Autodesk Fusion 360 part; units mm, degrees
(part 4 of 6)
  spline S7 degree 5 poles (100.0499, 27.0485) (100.0462, 27.0591) (100.039, 27.0805) (100.028, 27.1124) (100.0132, 27.1549) (99.9945, 27.2079) (99.9756, 27.2608) (99.9566, 27.3135) (99.9373, 27.366) (99.9178, 27.4184) (99.8981, 27.4707) (99.8782, 27.5228) (99.858, 27.5747) (99.8377, 27.6265) (99.8172, 27.6781) (99.7964, 27.7296) (99.7755, 27.7809) (99.7543, 27.832) (99.7329, 27.883) (99.7113, 27.9338) (99.6895, 27.9844) (99.6674, 28.0349) (99.6452, 28.0852) (99.6227, 28.1353) (99.6, 28.1852) (99.5771, 28.235) (99.554, 28.2846) (99.5307, 28.334) (99.5071, 28.3832) (99.4833, 28.4322) (99.4593, 28.481) (99.435, 28.5297) (99.4105, 28.5781) (99.3858, 28.6263) (99.3609, 28.6744) (99.3357, 28.7222) (99.3103, 28.7698) (99.2846, 28.8173) (99.2587, 28.8645) (99.2326, 28.9115) (99.2062, 28.9582) (99.1796, 29.0048) (99.1527, 29.0511) (99.1256, 29.0972) (99.0982, 29.143) (99.0706, 29.1886) (99.0427, 29.234) (99.0146, 29.2791) (98.9862, 29.324) (98.9575, 29.3686) (98.9286, 29.4129) (98.8993, 29.457) (98.8698, 29.5007) (98.84, 29.5442) (98.8098, 29.5873) (98.7794, 29.6302) (98.7487, 29.6728) (98.7177, 29.7152) (98.6865, 29.7572) (98.655, 29.7989) (98.623, 29.8402) (98.5906, 29.8811) (98.5578, 29.9214) (98.5245, 29.9612) (98.4907, 30.0006) (98.4567, 30.0397) (98.4225, 30.0785) (98.388, 30.1171) (98.3533, 30.1553) (98.3179, 30.1928) (98.2816, 30.2292) (98.2515, 30.2572) (98.2282, 30.2774) (98.2123, 30.2904) (98.2043, 30.2969) knots -1 -1 -1 -1 -1 -1 -0.98571429 -0.97142857 -0.95714286 -0.94285714 -0.92857143 -0.91428571 -0.9 -0.88571429 -0.87142857 -0.85714286 -0.84285714 -0.82857143 -0.81428571 -0.8 -0.78571429 -0.77142857 -0.75714286 -0.74285714 -0.72857143 -0.71428571 -0.7 -0.68571429 -0.67142857 -0.65714286 -0.64285714 -0.62857143 -0.61428571 -0.6 -0.58571429 -0.57142857 -0.55714286 -0.54285714 -0.52857143 -0.51428571 -0.5 -0.48571429 -0.47142857 -0.45714286 -0.44285714 -0.42857143 -0.41428571 -0.4 -0.38571429 -0.37142857 -0.35714286 -0.34285714 -0.32857143 -0.31428571 -0.3 -0.28571429 -0.27142857 -0.25714286 -0.24285714 -0.22857143 -0.21428571 -0.2 -0.18571429 -0.17142857 -0.15714286 -0.14285714 -0.12857143 -0.11428571 -0.1 -0.08571429 -0.07142857 -0.05714286 -0.04285714 -0.02857143 -0.01428571 0 0 0 0 0 0
  line L7 (98.2043, 30.2969) -> (97.816, 30.6089)
  arc A17 (97.7326, 31.303) -> (97.816, 30.6089) centre (98.1293, 30.9987) ccw
  arc A18 (97.7326, 31.303) -> (98.4247, 32.2557) centre (79.882, 45) ccw
  arc A19 (99.1106, 32.3908) -> (98.4247, 32.2557) centre (98.8368, 31.9725) ccw
  line L8 (99.1106, 32.3908) -> (99.5274, 32.118)
  spline S8 degree 5 poles (99.5274, 32.118) (99.536, 32.1123) (99.5534, 32.1013) (99.5797, 32.0854) (99.6156, 32.0654) (99.6615, 32.0421) (99.7081, 32.0201) (99.7552, 31.9988) (99.8025, 31.978) (99.85, 31.9574) (99.8977, 31.9371) (99.9456, 31.9172) (99.9938, 31.8978) (100.0423, 31.8791) (100.0911, 31.8609) (100.1403, 31.8433) (100.1897, 31.8261) (100.2393, 31.8094) (100.2892, 31.7931) (100.3392, 31.777) (100.3893, 31.7614) (100.4397, 31.746) (100.4902, 31.7311) (100.541, 31.7165) (100.5919, 31.7023) (100.643, 31.6885) (100.6943, 31.675) (100.7458, 31.6619) (100.7974, 31.6491) (100.8492, 31.6366) (100.9011, 31.6244) (100.9531, 31.6125) (101.0053, 31.6009) (101.0577, 31.5897) (101.1102, 31.5788) (101.1628, 31.5681) (101.2156, 31.5578) (101.2685, 31.5478) (101.3215, 31.538) (101.3746, 31.5286) (101.4279, 31.5194) (101.4813, 31.5105) (101.5348, 31.5019) (101.5884, 31.4936) (101.6422, 31.4856) (101.6961, 31.4778) (101.75, 31.4703) (101.8041, 31.4631) (101.8583, 31.4562) (101.9126, 31.4495) (101.967, 31.4431) (102.0215, 31.4369) (102.0761, 31.4311) (102.1308, 31.4254) (102.1856, 31.4201) (102.2405, 31.415) (102.2955, 31.4101) (102.3506, 31.4055) (102.4058, 31.4012) (102.461, 31.3971) (102.5164, 31.3933) (102.5718, 31.3897) (102.6274, 31.3864) (102.683, 31.3833) (102.7387, 31.3805) (102.7945, 31.3779) (102.8503, 31.3755) (102.9063, 31.3734) (102.9623, 31.3715) (103.0184, 31.3699) (103.0746, 31.3685) (103.1196, 31.3676) (103.1533, 31.3671) (103.1759, 31.3667) (103.1872, 31.3666) knots 0 0 0 0 0 0 0.01428571 0.02857143 0.04285714 0.05714286 0.07142857 0.08571429 0.1 0.11428571 0.12857143 0.14285714 0.15714286 0.17142857 0.18571429 0.2 0.21428571 0.22857143 0.24285714 0.25714286 0.27142857 0.28571429 0.3 0.31428571 0.32857143 0.34285714 0.35714286 0.37142857 0.38571429 0.4 0.41428571 0.42857143 0.44285714 0.45714286 0.47142857 0.48571429 0.5 0.51428571 0.52857143 0.54285714 0.55714286 0.57142857 0.58571429 0.6 0.61428571 0.62857143 0.64285714 0.65714286 0.67142857 0.68571429 0.7 0.71428571 0.72857143 0.74285714 0.75714286 0.77142857 0.78571429 0.8 0.81428571 0.82857143 0.84285714 0.85714286 0.87142857 0.88571429 0.9 0.91428571 0.92857143 0.94285714 0.95714286 0.97142857 0.98571429 1 1 1 1 1 1
  arc A20 (103.1872, 31.3666) -> (103.8806, 32.628) centre (79.882, 45) ccw
  spline S9 degree 5 poles (103.8806, 32.628) (103.8745, 32.6374) (103.8621, 32.6563) (103.8435, 32.6845) (103.8186, 32.722) (103.7874, 32.7687) (103.7559, 32.8152) (103.7243, 32.8615) (103.6926, 32.9076) (103.6607, 32.9535) (103.6286, 32.9992) (103.5964, 33.0447) (103.564, 33.09) (103.5314, 33.1351) (103.4987, 33.18) (103.4658, 33.2247) (103.4327, 33.2692) (103.3995, 33.3134) (103.3661, 33.3575) (103.3325, 33.4013) (103.2988, 33.4449) (103.2649, 33.4883) (103.2308, 33.5315) (103.1966, 33.5745) (103.1622, 33.6172) (103.1277, 33.6597) (103.0929, 33.7019) (103.058, 33.744) (103.023, 33.7858) (102.9877, 33.8273) (102.9523, 33.8687) (102.9167, 33.9097) (102.881, 33.9506) (102.845, 33.9911) (102.8089, 34.0315) (102.7726, 34.0715) (102.7362, 34.1113) (102.6995, 34.1509) (102.6627, 34.1902) (102.6257, 34.2292) (102.5886, 34.2679) (102.5512, 34.3064) (102.5137, 34.3446) (102.4759, 34.3825) (102.438, 34.4201) (102.3999, 34.4574) (102.3616, 34.4944) (102.3231, 34.5311) (102.2845, 34.5675) (102.2456, 34.6036) (102.2065, 34.6393) (102.1673, 34.6747) (102.1278, 34.7098) (102.0881, 34.7444) (102.0481, 34.7787) (102.008, 34.8127) (101.9677, 34.8463) (101.9272, 34.8796) (101.8865, 34.9126) (101.8455, 34.9451) (101.8043, 34.9772) (101.7628, 35.0087) (101.7209, 35.0396) (101.6788, 35.0699) (101.6363, 35.0997) (101.5936, 35.129) (101.5508, 35.1581) (101.5079, 35.1869) (101.4647, 35.2152) (101.4211, 35.2428) (101.3769, 35.2691) (101.3408, 35.2887) (101.3132, 35.3024) (101.2946, 35.3111) (101.2852, 35.3154) knots -1 -1 -1 -1 -1 -1 -0.98571429 -0.97142857 -0.95714286 -0.94285714 -0.92857143 -0.91428571 -0.9 -0.88571429 -0.87142857 -0.85714286 -0.84285714 -0.82857143 -0.81428571 -0.8 -0.78571429 -0.77142857 -0.75714286 -0.74285714 -0.72857143 -0.71428571 -0.7 -0.68571429 -0.67142857 -0.65714286 -0.64285714 -0.62857143 -0.61428571 -0.6 -0.58571429 -0.57142857 -0.55714286 -0.54285714 -0.52857143 -0.51428571 -0.5 -0.48571429 -0.47142857 -0.45714286 -0.44285714 -0.42857143 -0.41428571 -0.4 -0.38571429 -0.37142857 -0.35714286 -0.34285714 -0.32857143 -0.31428571 -0.3 -0.28571429 -0.27142857 -0.25714286 -0.24285714 -0.22857143 -0.21428571 -0.2 -0.18571429 -0.17142857 -0.15714286 -0.14285714 -0.12857143 -0.11428571 -0.1 -0.08571429 -0.07142857 -0.05714286 -0.04285714 -0.02857143 -0.01428571 0 0 0 0 0 0
  line L9 (101.2852, 35.3154) -> (100.8315, 35.5211)
  arc A21 (100.5781, 36.1726) -> (100.8315, 35.5211) centre (101.038, 35.9765) ccw
  arc A22 (100.5781, 36.1726) -> (101.0116, 37.2674) centre (79.882, 45) ccw
  arc A23 (101.6423, 37.5689) -> (101.0116, 37.2674) centre (101.4811, 37.0956) ccw
  line L10 (101.6423, 37.5689) -> (102.1139, 37.4083)
  spline S10 degree 5 poles (102.1139, 37.4083) (102.1236, 37.405) (102.1431, 37.3986) (102.1726, 37.3897) (102.2124, 37.3793) (102.2626, 37.3682) (102.3132, 37.3584) (102.3641, 37.3495) (102.4151, 37.3411) (102.4662, 37.333) (102.5175, 37.3252) (102.5688, 37.3178) (102.6203, 37.311) (102.6719, 37.3049) (102.7238, 37.2995) (102.7758, 37.2946) (102.8279, 37.2903) (102.8801, 37.2865) (102.9325, 37.283) (102.9849, 37.28) (103.0374, 37.2772) (103.09, 37.2749) (103.1426, 37.273) (103.1954, 37.2715) (103.2483, 37.2704) (103.3012, 37.2697) (103.3543, 37.2695) (103.4074, 37.2695) (103.4605, 37.2699) (103.5138, 37.2707) (103.5671, 37.2718) (103.6205, 37.2733) (103.6739, 37.275) (103.7274, 37.2772) (103.781, 37.2796) (103.8346, 37.2824) (103.8883, 37.2855) (103.942, 37.289) (103.9958, 37.2927) (104.0496, 37.2968) (104.1035, 37.3012) (104.1574, 37.3059) (104.2114, 37.3108) (104.2654, 37.3161) (104.3195, 37.3217) (104.3736, 37.3276) (104.4277, 37.3337) (104.4819, 37.3402) (104.5361, 37.347) (104.5903, 37.354) (104.6446, 37.3613) (104.699, 37.3689) (104.7533, 37.3768) (104.8077, 37.385) (104.8621, 37.3934) (104.9165, 37.4021) (104.971, 37.4111) (105.0255, 37.4203) (105.08, 37.4299) (105.1346, 37.4397) (105.1892, 37.4497) (105.2437, 37.46) (105.2984, 37.4706) (105.353, 37.4815) (105.4077, 37.4926) (105.4623, 37.5039) (105.517, 37.5155) (105.5717, 37.5274) (105.6264, 37.5395) (105.6812, 37.5519) (105.7359, 37.5646) (105.7797, 37.5749) (105.8126, 37.5827) (105.8345, 37.588) (105.8455, 37.5906) knots 0 0 0 0 0 0 0.01428571 0.02857143 0.04285714 0.05714286 0.07142857 0.08571429 0.1 0.11428571 0.12857143 0.14285714 0.15714286 0.17142857 0.18571429 0.2 0.21428571 0.22857143 0.24285714 0.25714286 0.27142857 0.28571429 0.3 0.31428571 0.32857143 0.34285714 0.35714286 0.37142857 0.38571429 0.4 0.41428571 0.42857143 0.44285714 0.45714286 0.47142857 0.48571429 0.5 0.51428571 0.52857143 0.54285714 0.55714286 0.57142857 0.58571429 0.6 0.61428571 0.62857143 0.64285714 0.65714286 0.67142857 0.68571429 0.7 0.71428571 0.72857143 0.74285714 0.75714286 0.77142857 0.78571429 0.8 0.81428571 0.82857143 0.84285714 0.85714286 0.87142857 0.88571429 0.9 0.91428571 0.92857143 0.94285714 0.95714286 0.97142857 0.98571429 1 1 1 1 1 1
  arc A24 (105.8455, 37.5906) -> (106.2035, 38.9849) centre (79.882, 45) ccw
  spline S11 degree 5 poles (106.2035, 38.9849) (106.1951, 38.9925) (106.1785, 39.0077) (106.1535, 39.0304) (106.12, 39.0605) (106.0781, 39.098) (106.0361, 39.1352) (105.994, 39.1722) (105.9518, 39.2089) (105.9095, 39.2455) (105.867, 39.2817) (105.8245, 39.3178) (105.7818, 39.3536) (105.7391, 39.3892) (105.6962, 39.4246) (105.6532, 39.4597) (105.6101, 39.4945) (105.567, 39.5291) (105.5237, 39.5635) (105.4803, 39.5976) (105.4367, 39.6315) (105.3931, 39.6651) (105.3494, 39.6984) (105.3056, 39.7315) (105.2616, 39.7643) (105.2176, 39.7969) (105.1734, 39.8292) (105.1292, 39.8612) (105.0848, 39.893) (105.0403, 39.9245) (104.9958, 39.9557) (104.9511, 39.9867) (104.9063, 40.0173) (104.8614, 40.0477) (104.8164, 40.0778) (104.7713, 40.1075) (104.7261, 40.137) (104.6807, 40.1662) (104.6353, 40.1951) (104.5898, 40.2237) (104.5441, 40.252) (104.4984, 40.28) (104.4525, 40.3076) (104.4066, 40.3349) (104.3605, 40.3619) (104.3143, 40.3885) (104.268, 40.4149) (104.2216, 40.4408) (104.1751, 40.4665) (104.1285, 40.4918) (104.0818, 40.5167) (104.0349, 40.5412) (103.988, 40.5653) (103.9409, 40.589) (103.8937, 40.6123) (103.8464, 40.6352) (103.7989, 40.6578) (103.7514, 40.68) (103.7038, 40.7018) (103.656, 40.7231) (103.6082, 40.7439) (103.5601, 40.7641) (103.5119, 40.7836) (103.4635, 40.8025) (103.415, 40.8208) (103.3663, 40.8386) (103.3176, 40.8561) (103.2689, 40.8733) (103.22, 40.89) (103.1709, 40.9059) (103.1216, 40.9203) (103.0817, 40.9303) (103.0516, 40.9368) (103.0314, 40.9406) (103.0213, 40.9424) knots -1 -1 -1 -1 -1 -1 -0.98571429 -0.97142857 -0.95714286 -0.94285714 -0.92857143 -0.91428571 -0.9 -0.88571429 -0.87142857 -0.85714286 -0.84285714 -0.82857143 -0.81428571 -0.8 -0.78571429 -0.77142857 -0.75714286 -0.74285714 -0.72857143 -0.71428571 -0.7 -0.68571429 -0.67142857 -0.65714286 -0.64285714 -0.62857143 -0.61428571 -0.6 -0.58571429 -0.57142857 -0.55714286 -0.54285714 -0.52857143 -0.51428571 -0.5 -0.48571429 -0.47142857 -0.45714286 -0.44285714 -0.42857143 -0.41428571 -0.4 -0.38571429 -0.37142857 -0.35714286 -0.34285714 -0.32857143 -0.31428571 -0.3 -0.28571429 -0.27142857 -0.25714286 -0.24285714 -0.22857143 -0.21428571 -0.2 -0.18571429 -0.17142857 -0.15714286 -0.14285714 -0.12857143 -0.11428571 -0.1 -0.08571429 -0.07142857 -0.05714286 -0.04285714 -0.02857143 -0.01428571 0 0 0 0 0 0
  line L11 (103.0213, 40.9424) -> (102.5307, 41.0288)
  arc A25 (102.1232, 41.5969) -> (102.5307, 41.0288) centre (102.6174, 41.5212) ccw
  arc A26 (102.1232, 41.5969) -> (102.2707, 42.7651) centre (79.882, 45) ccw
  arc A27 (102.8067, 43.2139) -> (102.2707, 42.7651) centre (102.7683, 42.7154) ccw
  line L12 (102.8067, 43.2139) -> (103.3034, 43.1756)
  spline S12 degree 5 poles (103.3034, 43.1756) (103.3136, 43.1748) (103.3342, 43.1735) (103.3649, 43.1723) (103.406, 43.1721) (103.4574, 43.1738) (103.5089, 43.1769) (103.5604, 43.181) (103.6119, 43.1855) (103.6634, 43.1903) (103.715, 43.1955) (103.7665, 43.2012) (103.8181, 43.2074) (103.8696, 43.2143) (103.9212, 43.2219) (103.9728, 43.2302) (104.0243, 43.239) (104.0759, 43.2482) (104.1274, 43.2579) (104.1789, 43.2679) (104.2305, 43.2784) (104.282, 43.2892) (104.3335, 43.3004) (104.385, 43.3121) (104.4364, 43.3242) (104.4879, 43.3367) (104.5393, 43.3496) (104.5908, 43.3629) (104.6422, 43.3765) (104.6935, 43.3905) (104.7449, 43.4048) (104.7962, 43.4195) (104.8476, 43.4345) (104.8989, 43.4499) (104.9501, 43.4656) (105.0014, 43.4816) (105.0526, 43.498) (105.1038, 43.5147) (105.1549, 43.5317) (105.206, 43.549) (105.2571, 43.5667) (105.3082, 43.5846) (105.3592, 43.6029) (105.4103, 43.6214) (105.4612, 43.6403) (105.5122, 43.6594) (105.5631, 43.6789) (105.6139, 43.6986) (105.6648, 43.7186) (105.7156, 43.7389) (105.7663, 43.7595) (105.8171, 43.7804) (105.8677, 43.8015) (105.9184, 43.823) (105.969, 43.8447) (106.0196, 43.8666) (106.0701, 43.8889) (106.1206, 43.9114) (106.171, 43.9342) (106.2214, 43.9572) (106.2718, 43.9806) (106.3221, 44.0041) (106.3723, 44.028) (106.4226, 44.052) (106.4727, 44.0764) (106.5229, 44.101) (106.573, 44.1258) (106.623, 44.151) (106.673, 44.1763) (106.7229, 44.2019) (106.7728, 44.2278) (106.8127, 44.2486) (106.8426, 44.2644) (106.8625, 44.275) (106.8724, 44.2803) knots 0 0 0 0 0 0 0.01428571 0.02857143 0.04285714 0.05714286 0.07142857 0.08571429 0.1 0.11428571 0.12857143 0.14285714 0.15714286 0.17142857 0.18571429 0.2 0.21428571 0.22857143 0.24285714 0.25714286 0.27142857 0.28571429 0.3 0.31428571 0.32857143 0.34285714 0.35714286 0.37142857 0.38571429 0.4 0.41428571 0.42857143 0.44285714 0.45714286 0.47142857 0.48571429 0.5 0.51428571 0.52857143 0.54285714 0.55714286 0.57142857 0.58571429 0.6 0.61428571 0.62857143 0.64285714 0.65714286 0.67142857 0.68571429 0.7 0.71428571 0.72857143 0.74285714 0.75714286 0.77142857 0.78571429 0.8 0.81428571 0.82857143 0.84285714 0.85714286 0.87142857 0.88571429 0.9 0.91428571 0.92857143 0.94285714 0.95714286 0.97142857 0.98571429 1 1 1 1 1 1
  arc A28 (106.8724, 44.2803) -> (106.8724, 45.7197) centre (79.882, 45) ccw
  spline S13 degree 5 poles (106.8724, 45.7197) (106.8625, 45.725) (106.8426, 45.7356) (106.8127, 45.7514) (106.7728, 45.7722) (106.7229, 45.7981) (106.673, 45.8237) (106.623, 45.849) (106.573, 45.8742) (106.5229, 45.899) (106.4727, 45.9236) (106.4226, 45.948) (106.3723, 45.972) (106.3221, 45.9959) (106.2718, 46.0194) (106.2214, 46.0428) (106.171, 46.0658) (106.1206, 46.0886) (106.0701, 46.1111) (106.0196, 46.1334) (105.969, 46.1553) (105.9184, 46.177) (105.8677, 46.1985) (105.8171, 46.2196) (105.7663, 46.2405) (105.7156, 46.2611) (105.6648, 46.2814) (105.6139, 46.3014) (105.5631, 46.3211) (105.5122, 46.3406) (105.4612, 46.3597) (105.4103, 46.3786) (105.3592, 46.3971) (105.3082, 46.4154) (105.2571, 46.4333) (105.206, 46.451) (105.1549, 46.4683) (105.1038, 46.4853) (105.0526, 46.502) (105.0014, 46.5184) (104.9501, 46.5344) (104.8989, 46.5501) (104.8476, 46.5655) (104.7962, 46.5805) (104.7449, 46.5952) (104.6935, 46.6095) (104.6422, 46.6235) (104.5908, 46.6371) (104.5393, 46.6504) (104.4879, 46.6633) (104.4364, 46.6758) (104.385, 46.6879) (104.3335, 46.6996) (104.282, 46.7108) (104.2305, 46.7216) (104.1789, 46.7321) (104.1274, 46.7421) (104.0759, 46.7518) (104.0243, 46.761) (103.9728, 46.7698) (103.9212, 46.7781) (103.8696, 46.7857) (103.8181, 46.7926) (103.7665, 46.7988) (103.715, 46.8045) (103.6634, 46.8097) (103.6119, 46.8145) (103.5604, 46.819) (103.5089, 46.8231) (103.4574, 46.8262) (103.406, 46.8279) (103.3649, 46.8277) (103.3342, 46.8265) (103.3136, 46.8252) (103.3034, 46.8244) knots -1 -1 -1 -1 -1 -1 -0.98571429 -0.97142857 -0.95714286 -0.94285714 -0.92857143 -0.91428571 -0.9 -0.88571429 -0.87142857 -0.85714286 -0.84285714 -0.82857143 -0.81428571 -0.8 -0.78571429 -0.77142857 -0.75714286 -0.74285714 -0.72857143 -0.71428571 -0.7 -0.68571429 -0.67142857 -0.65714286 -0.64285714 -0.62857143 -0.61428571 -0.6 -0.58571429 -0.57142857 -0.55714286 -0.54285714 -0.52857143 -0.51428571 -0.5 -0.48571429 -0.47142857 -0.45714286 -0.44285714 -0.42857143 -0.41428571 -0.4 -0.38571429 -0.37142857 -0.35714286 -0.34285714 -0.32857143 -0.31428571 -0.3 -0.28571429 -0.27142857 -0.25714286 -0.24285714 -0.22857143 -0.21428571 -0.2 -0.18571429 -0.17142857 -0.15714286 -0.14285714 -0.12857143 -0.11428571 -0.1 -0.08571429 -0.07142857 -0.05714286 -0.04285714 -0.02857143 -0.01428571 0 0 0 0 0 0
  line L13 (103.3034, 46.8244) -> (102.8067, 46.7861)
  arc A29 (102.2707, 47.2349) -> (102.8067, 46.7861) centre (102.7683, 47.2846) ccw
  arc A30 (102.2707, 47.2349) -> (102.1232, 48.4031) centre (79.882, 45) ccw
  arc A31 (102.5307, 48.9712) -> (102.1232, 48.4031) centre (102.6174, 48.4788) ccw
  line L14 (102.5307, 48.9712) -> (103.0213, 49.0576)
  spline S14 degree 5 poles (103.0213, 49.0576) (103.0314, 49.0594) (103.0516, 49.0632) (103.0817, 49.0697) (103.1216, 49.0797) (103.1709, 49.0941) (103.22, 49.11) (103.2689, 49.1267) (103.3176, 49.1439) (103.3663, 49.1614) (103.415, 49.1792) (103.4635, 49.1975) (103.5119, 49.2164) (103.5601, 49.2359) (103.6082, 49.2561) (103.656, 49.2769) (103.7038, 49.2982) (103.7514, 49.32) (103.7989, 49.3422) (103.8464, 49.3648) (103.8937, 49.3877) (103.9409, 49.411) (103.988, 49.4347) (104.0349, 49.4588) (104.0818, 49.4833) (104.1285, 49.5082) (104.1751, 49.5335) (104.2216, 49.5592) (104.268, 49.5851) (104.3143, 49.6115) (104.3605, 49.6381) (104.4066, 49.6651) (104.4525, 49.6924) (104.4984, 49.72) (104.5441, 49.748) (104.5898, 49.7763) (104.6353, 49.8049) (104.6807, 49.8338) (104.7261, 49.863) (104.7713, 49.8925) (104.8164, 49.9222) (104.8614, 49.9523) (104.9063, 49.9827) (104.9511, 50.0133) (104.9958, 50.0443) (105.0403, 50.0755) (105.0848, 50.107) (105.1292, 50.1388) (105.1734, 50.1708) (105.2176, 50.2031) (105.2616, 50.2357) (105.3056, 50.2685) (105.3494, 50.3016) (105.3931, 50.3349) (105.4367, 50.3685) (105.4803, 50.4024) (105.5237, 50.4365) (105.567, 50.4709) (105.6101, 50.5055) (105.6532, 50.5403) (105.6962, 50.5754) (105.7391, 50.6108) (105.7818, 50.6464) (105.8245, 50.6822) (105.867, 50.7183) (105.9095, 50.7545) (105.9518, 50.7911) (105.994, 50.8278) (106.0361, 50.8648) (106.0781, 50.902) (106.12, 50.9395) (106.1535, 50.9696) (106.1785, 50.9923) (106.1951, 51.0075) (106.2035, 51.0151) knots 0 0 0 0 0 0 0.01428571 0.02857143 0.04285714 0.05714286 0.07142857 0.08571429 0.1 0.11428571 0.12857143 0.14285714 0.15714286 0.17142857 0.18571429 0.2 0.21428571 0.22857143 0.24285714 0.25714286 0.27142857 0.28571429 0.3 0.31428571 0.32857143 0.34285714 0.35714286 0.37142857 0.38571429 0.4 0.41428571 0.42857143 0.44285714 0.45714286 0.47142857 0.48571429 0.5 0.51428571 0.52857143 0.54285714 0.55714286 0.57142857 0.58571429 0.6 0.61428571 0.62857143 0.64285714 0.65714286 0.67142857 0.68571429 0.7 0.71428571 0.72857143 0.74285714 0.75714286 0.77142857 0.78571429 0.8 0.81428571 0.82857143 0.84285714 0.85714286 0.87142857 0.88571429 0.9 0.91428571 0.92857143 0.94285714 0.95714286 0.97142857 0.98571429 1 1 1 1 1 1
  arc A32 (106.2035, 51.0151) -> (105.8455, 52.4094) centre (79.882, 45) ccw
  spline S15 degree 5 poles (105.8455, 52.4094) (105.8345, 52.412) (105.8126, 52.4173) (105.7797, 52.4251) (105.7359, 52.4354) (105.6812, 52.4481) (105.6264, 52.4605) (105.5717, 52.4726) (105.517, 52.4845) (105.4623, 52.4961) (105.4077, 52.5074) (105.353, 52.5185) (105.2984, 52.5294) (105.2437, 52.54) (105.1892, 52.5503) (105.1346, 52.5603) (105.08, 52.5701) (105.0255, 52.5797) (104.971, 52.5889) (104.9165, 52.5979) (104.8621, 52.6066) (104.8077, 52.615) (104.7533, 52.6232) (104.699, 52.6311) (104.6446, 52.6387) (104.5903, 52.646) (104.5361, 52.653) (104.4819, 52.6598) (104.4277, 52.6663) (104.3736, 52.6724) (104.3195, 52.6783) (104.2654, 52.6839) (104.2114, 52.6892) (104.1574, 52.6941) (104.1035, 52.6988) (104.0496, 52.7032) (103.9958, 52.7073) (103.942, 52.711) (103.8883, 52.7145) (103.8346, 52.7176) (103.781, 52.7204) (103.7274, 52.7228) (103.6739, 52.725) (103.6205, 52.7267) (103.5671, 52.7282) (103.5138, 52.7293) (103.4605, 52.7301) (103.4074, 52.7305) (103.3543, 52.7305) (103.3012, 52.7303) (103.2483, 52.7296) (103.1954, 52.7285) (103.1426, 52.727) (103.09, 52.7251) (103.0374, 52.7228) (102.9849, 52.72) (102.9325, 52.717) (102.8801, 52.7135) (102.8279, 52.7097) (102.7758, 52.7054) (102.7238, 52.7005) (102.6719, 52.6951) (102.6203, 52.689) (102.5688, 52.6822) (102.5175, 52.6748) (102.4662, 52.667) (102.4151, 52.6589) (102.3641, 52.6505) (102.3132, 52.6416) (102.2626, 52.6318) (102.2124, 52.6207) (102.1726, 52.6103) (102.1431, 52.6014) (102.1236, 52.595) (102.1139, 52.5917) knots -1 -1 -1 -1 -1 -1 -0.98571429 -0.97142857 -0.95714286 -0.94285714 -0.92857143 -0.91428571 -0.9 -0.88571429 -0.87142857 -0.85714286 -0.84285714 -0.82857143 -0.81428571 -0.8 -0.78571429 -0.77142857 -0.75714286 -0.74285714 -0.72857143 -0.71428571 -0.7 -0.68571429 -0.67142857 -0.65714286 -0.64285714 -0.62857143 -0.61428571 -0.6 -0.58571429 -0.57142857 -0.55714286 -0.54285714 -0.52857143 -0.51428571 -0.5 -0.48571429 -0.47142857 -0.45714286 -0.44285714 -0.42857143 -0.41428571 -0.4 -0.38571429 -0.37142857 -0.35714286 -0.34285714 -0.32857143 -0.31428571 -0.3 -0.28571429 -0.27142857 -0.25714286 -0.24285714 -0.22857143 -0.21428571 -0.2 -0.18571429 -0.17142857 -0.15714286 -0.14285714 -0.12857143 -0.11428571 -0.1 -0.08571429 -0.07142857 -0.05714286 -0.04285714 -0.02857143 -0.01428571 0 0 0 0 0 0
  line L15 (102.1139, 52.5917) -> (101.6423, 52.4311)
  arc A33 (101.0116, 52.7326) -> (101.6423, 52.4311) centre (101.4811, 52.9044) ccw
  arc A34 (101.0116, 52.7326) -> (100.5781, 53.8274) centre (79.882, 45) ccw
  arc A35 (100.8315, 54.4789) -> (100.5781, 53.8274) centre (101.038, 54.0235) ccw
  line L16 (100.8315, 54.4789) -> (101.2852, 54.6846)
  spline S16 degree 5 poles (101.2852, 54.6846) (101.2946, 54.6889) (101.3132, 54.6976) (101.3408, 54.7113) (101.3769, 54.7309) (101.4211, 54.7572) (101.4647, 54.7848) (101.5079, 54.8131) (101.5508, 54.8419) (101.5936, 54.871) (101.6363, 54.9003) (101.6788, 54.9301) (101.7209, 54.9604) (101.7628, 54.9913) (101.8043, 55.0228) (101.8455, 55.0549) (101.8865, 55.0874) (101.9272, 55.1204) (101.9677, 55.1537) (102.008, 55.1873) (102.0481, 55.2213) (102.0881, 55.2556) (102.1278, 55.2902) (102.1673, 55.3253) (102.2065, 55.3607) (102.2456, 55.3964) (102.2845, 55.4325) (102.3231, 55.4689) (102.3616, 55.5056) (102.3999, 55.5426) (102.438, 55.5799) (102.4759, 55.6175) (102.5137, 55.6554) (102.5512, 55.6936) (102.5886, 55.7321) (102.6257, 55.7708) (102.6627, 55.8098) (102.6995, 55.8491) (102.7362, 55.8887) (102.7726, 55.9285) (102.8089, 55.9685) (102.845, 56.0089) (102.881, 56.0494) (102.9167, 56.0903) (102.9523, 56.1313) (102.9877, 56.1727) (103.023, 56.2142) (103.058, 56.256) (103.0929, 56.2981) (103.1277, 56.3403) (103.1622, 56.3828) (103.1966, 56.4255) (103.2308, 56.4685) (103.2649, 56.5117) (103.2988, 56.5551) (103.3325, 56.5987) (103.3661, 56.6425) (103.3995, 56.6866) (103.4327, 56.7308) (103.4658, 56.7753) (103.4987, 56.82) (103.5314, 56.8649) (103.564, 56.91) (103.5964, 56.9553) (103.6286, 57.0008) (103.6607, 57.0465) (103.6926, 57.0924) (103.7243, 57.1385) (103.7559, 57.1848) (103.7874, 57.2313) (103.8186, 57.278) (103.8435, 57.3155) (103.8621, 57.3437) (103.8745, 57.3626) (103.8806, 57.372) knots 0 0 0 0 0 0 0.01428571 0.02857143 0.04285714 0.05714286 0.07142857 0.08571429 0.1 0.11428571 0.12857143 0.14285714 0.15714286 0.17142857 0.18571429 0.2 0.21428571 0.22857143 0.24285714 0.25714286 0.27142857 0.28571429 0.3 0.31428571 0.32857143 0.34285714 0.35714286 0.37142857 0.38571429 0.4 0.41428571 0.42857143 0.44285714 0.45714286 0.47142857 0.48571429 0.5 0.51428571 0.52857143 0.54285714 0.55714286 0.57142857 0.58571429 0.6 0.61428571 0.62857143 0.64285714 0.65714286 0.67142857 0.68571429 0.7 0.71428571 0.72857143 0.74285714 0.75714286 0.77142857 0.78571429 0.8 0.81428571 0.82857143 0.84285714 0.85714286 0.87142857 0.88571429 0.9 0.91428571 0.92857143 0.94285714 0.95714286 0.97142857 0.98571429 1 1 1 1 1 1
  arc A36 (103.8806, 57.372) -> (103.1872, 58.6334) centre (79.882, 45) ccw
  spline S17 degree 5 poles (103.1872, 58.6334) (103.1759, 58.6333) (103.1533, 58.6329) (103.1196, 58.6324) (103.0746, 58.6315) (103.0184, 58.6301) (102.9623, 58.6285) (102.9063, 58.6266) (102.8503, 58.6245) (102.7945, 58.6221) (102.7387, 58.6195) (102.683, 58.6167) (102.6274, 58.6136) (102.5718, 58.6103) (102.5164, 58.6067) (102.461, 58.6029) (102.4058, 58.5988) (102.3506, 58.5945) (102.2955, 58.5899) (102.2405, 58.585) (102.1856, 58.5799) (102.1308, 58.5746) (102.0761, 58.5689) (102.0215, 58.5631) (101.967, 58.5569) (101.9126, 58.5505) (101.8583, 58.5438) (101.8041, 58.5369) (101.75, 58.5297) (101.6961, 58.5222) (101.6422, 58.5144) (101.5884, 58.5064) (101.5348, 58.4981) (101.4813, 58.4895) (101.4279, 58.4806) (101.3746, 58.4714) (101.3215, 58.462) (101.2685, 58.4522) (101.2156, 58.4422) (101.1628, 58.4319) (101.1102, 58.4212) (101.0577, 58.4103) (101.0053, 58.3991) (100.9531, 58.3875) (100.9011, 58.3756) (100.8492, 58.3634) (100.7974, 58.3509) (100.7458, 58.3381) (100.6943, 58.325) (100.643, 58.3115) (100.5919, 58.2977) (100.541, 58.2835) (100.4902, 58.2689) (100.4397, 58.254) (100.3893, 58.2386) (100.3392, 58.223) (100.2892, 58.2069) (100.2393, 58.1906) (100.1897, 58.1739) (100.1403, 58.1567) (100.0911, 58.1391) (100.0423, 58.1209) (99.9938, 58.1022) (99.9456, 58.0828) (99.8977, 58.0629) (99.85, 58.0426) (99.8025, 58.022) (99.7552, 58.0012) (99.7081, 57.9799) (99.6615, 57.9579) (99.6156, 57.9346) (99.5797, 57.9146) (99.5534, 57.8987) (99.536, 57.8877) (99.5274, 57.882) knots -1 -1 -1 -1 -1 -1 -0.98571429 -0.97142857 -0.95714286 -0.94285714 -0.92857143 -0.91428571 -0.9 -0.88571429 -0.87142857 -0.85714286 -0.84285714 -0.82857143 -0.81428571 -0.8 -0.78571429 -0.77142857 -0.75714286 -0.74285714 -0.72857143 -0.71428571 -0.7 -0.68571429 -0.67142857 -0.65714286 -0.64285714 -0.62857143 -0.61428571 -0.6 -0.58571429 -0.57142857 -0.55714286 -0.54285714 -0.52857143 -0.51428571 -0.5 -0.48571429 -0.47142857 -0.45714286 -0.44285714 -0.42857143 -0.41428571 -0.4 -0.38571429 -0.37142857 -0.35714286 -0.34285714 -0.32857143 -0.31428571 -0.3 -0.28571429 -0.27142857 -0.25714286 -0.24285714 -0.22857143 -0.21428571 -0.2 -0.18571429 -0.17142857 -0.15714286 -0.14285714 -0.12857143 -0.11428571 -0.1 -0.08571429 -0.07142857 -0.05714286 -0.04285714 -0.02857143 -0.01428571 0 0 0 0 0 0
  line L17 (99.5274, 57.882) -> (99.1106, 57.6092)
  arc A37 (98.4247, 57.7443) -> (99.1106, 57.6092) centre (98.8368, 58.0275) ccw
  arc A38 (98.4247, 57.7443) -> (98.0849, 58.2252) centre (79.882, 45) ccw
  line L18 (98.0849, 58.2252) -> (106.9873, 66.5851)
  arc A39 (111.7668, 69.0797) -> (106.9873, 66.5851) centre (113.8328, 59.2954) ccw
  arc A40 (111.7668, 69.0797) -> (105.9162, 75.3099) centre (110.7338, 73.9718) ccw
  arc A41 (103.1265, 70.6965) -> (105.9162, 75.3099) centre (96.281, 77.9862) ccw
  line L19 (103.1265, 70.6965) -> (94.2241, 62.3365)
  arc A42 (94.2241, 62.3365) -> (93.7655, 62.7059) centre (79.882, 45) ccw
  arc A43 (93.6737, 63.3989) -> (93.7655, 62.7059) centre (94.074, 63.0994) ccw
  line L20 (93.6737, 63.3989) -> (93.9722, 63.7978)
  spline S18 degree 5 poles (93.9722, 63.7978) (93.9783, 63.806) (93.9905, 63.8226) (94.008, 63.8479) (94.0302, 63.8825) (94.0563, 63.9268) (94.0812, 63.972) (94.1054, 64.0176) (94.1292, 64.0635) (94.1527, 64.1096) (94.1759, 64.1559) (94.1988, 64.2025) (94.2212, 64.2494) (94.2429, 64.2966) (94.2642, 64.3442) (94.2848, 64.3922) (94.305, 64.4404) (94.3248, 64.4889) (94.3443, 64.5376) (94.3634, 64.5865) (94.3822, 64.6356) (94.4007, 64.6849) (94.4188, 64.7344) (94.4365, 64.7841) (94.4539, 64.8341) (94.4709, 64.8842) (94.4875, 64.9346) (94.5039, 64.9851) (94.5199, 65.0358) (94.5356, 65.0867) (94.5511, 65.1377) (94.5662, 65.1889) (94.581, 65.2403) (94.5955, 65.2918) (94.6097, 65.3435) (94.6236, 65.3954) (94.6372, 65.4474) (94.6506, 65.4996) (94.6636, 65.5519) (94.6764, 65.6043) (94.6889, 65.6569) (94.7011, 65.7096) (94.713, 65.7625) (94.7247, 65.8155) (94.7361, 65.8687) (94.7472, 65.9219) (94.7581, 65.9753) (94.7687, 66.0289) (94.779, 66.0825) (94.7891, 66.1363) (94.7989, 66.1902) (94.8085, 66.2442) (94.8178, 66.2983) (94.8268, 66.3525) (94.8356, 66.4069) (94.8441, 66.4614) (94.8524, 66.516) (94.8605, 66.5706) (94.8683, 66.6254) (94.8758, 66.6803) (94.8831, 66.7354) (94.8902, 66.7905) (94.897, 66.8457) (94.9035, 66.901) (94.9099, 66.9564) (94.916, 67.0119) (94.9218, 67.0675) (94.9274, 67.1232) (94.9328, 67.179) (94.9379, 67.2349) (94.9428, 67.2909) (94.9466, 67.3357) (94.9493, 67.3694) (94.951, 67.3919) (94.9519, 67.4031) knots 0 0 0 0 0 0 0.01428571 0.02857143 0.04285714 0.05714286 0.07142857 0.08571429 0.1 0.11428571 0.12857143 0.14285714 0.15714286 0.17142857 0.18571429 0.2 0.21428571 0.22857143 0.24285714 0.25714286 0.27142857 0.28571429 0.3 0.31428571 0.32857143 0.34285714 0.35714286 0.37142857 0.38571429 0.4 0.41428571 0.42857143 0.44285714 0.45714286 0.47142857 0.48571429 0.5 0.51428571 0.52857143 0.54285714 0.55714286 0.57142857 0.58571429 0.6 0.61428571 0.62857143 0.64285714 0.65714286 0.67142857 0.68571429 0.7 0.71428571 0.72857143 0.74285714 0.75714286 0.77142857 0.78571429 0.8 0.81428571 0.82857143 0.84285714 0.85714286 0.87142857 0.88571429 0.9 0.91428571 0.92857143 0.94285714 0.95714286 0.97142857 0.98571429 1 1 1 1 1 1
  arc A44 (94.9519, 67.4031) -> (93.7365, 68.1744) centre (79.882, 45) ccw
  spline S19 degree 5 poles (93.7365, 68.1744) (93.7267, 68.1688) (93.7071, 68.1577) (93.6778, 68.1409) (93.6388, 68.1184) (93.5902, 68.0902) (93.5419, 68.0617) (93.4937, 68.0331) (93.4457, 68.0043) (93.3978, 67.9753) (93.3502, 67.9462) (93.3028, 67.9169) (93.2555, 67.8874) (93.2085, 67.8577) (93.1616, 67.8278) (93.1149, 67.7978) (93.0685, 67.7676) (93.0222, 67.7372) (92.9761, 67.7067) (92.9303, 67.6759) (92.8846, 67.645) (92.8392, 67.6139) (92.794, 67.5826) (92.749, 67.5512) (92.7042, 67.5195) (92.6596, 67.4877) (92.6152, 67.4557) (92.5711, 67.4235) (92.5271, 67.3911) (92.4834, 67.3586) (92.44, 67.3258) (92.3968, 67.2929) (92.3538, 67.2598) (92.311, 67.2264) (92.2685, 67.1929) (92.2262, 67.1592) (92.1842, 67.1254) (92.1424, 67.0913) (92.1009, 67.057) (92.0596, 67.0225) (92.0186, 66.9879) (91.9779, 66.953) (91.9375, 66.9179) (91.8973, 66.8826) (91.8574, 66.8472) (91.8178, 66.8115) (91.7784, 66.7756) (91.7394, 66.7395) (91.7006, 66.7032) (91.6622, 66.6667) (91.624, 66.6299) (91.5862, 66.5929) (91.5488, 66.5557) (91.5117, 66.5183) (91.4749, 66.4806) (91.4385, 66.4427) (91.4024, 66.4045) (91.3667, 66.3662) (91.3312, 66.3276) (91.2961, 66.2888) (91.2616, 66.2497) (91.2275, 66.2102) (91.194, 66.1704) (91.1612, 66.1302) (91.1288, 66.0897) (91.0968, 66.049) (91.0651, 66.0081) (91.0336, 65.967) (91.0027, 65.9257) (90.9724, 65.8839) (90.9434, 65.8414) (90.9216, 65.8066) (90.9061, 65.78) (90.8963, 65.7619) (90.8915, 65.7529) knots -1 -1 -1 -1 -1 -1 -0.98571429 -0.97142857 -0.95714286 -0.94285714 -0.92857143 -0.91428571 -0.9 -0.88571429 -0.87142857 -0.85714286 -0.84285714 -0.82857143 -0.81428571 -0.8 -0.78571429 -0.77142857 -0.75714286 -0.74285714 -0.72857143 -0.71428571 -0.7 -0.68571429 -0.67142857 -0.65714286 -0.64285714 -0.62857143 -0.61428571 -0.6 -0.58571429 -0.57142857 -0.55714286 -0.54285714 -0.52857143 -0.51428571 -0.5 -0.48571429 -0.47142857 -0.45714286 -0.44285714 -0.42857143 -0.41428571 -0.4 -0.38571429 -0.37142857 -0.35714286 -0.34285714 -0.32857143 -0.31428571 -0.3 -0.28571429 -0.27142857 -0.25714286 -0.24285714 -0.22857143 -0.21428571 -0.2 -0.18571429 -0.17142857 -0.15714286 -0.14285714 -0.12857143 -0.11428571 -0.1 -0.08571429 -0.07142857 -0.05714286 -0.04285714 -0.02857143 -0.01428571 0 0 0 0 0 0
  line L21 (90.8915, 65.7529) -> (90.6577, 65.313)
  arc A45 (89.9915, 65.101) -> (90.6577, 65.313) centre (90.2161, 65.5476) ccw
  arc A46 (89.9915, 65.101) -> (88.926, 65.6023) centre (79.882, 45) ccw
  arc A47 (88.6648, 66.2508) -> (88.926, 65.6023) centre (89.127, 66.0601) ccw
  line L22 (88.6648, 66.2508) -> (88.8547, 66.7113)
  spline S20 degree 5 poles (88.8547, 66.7113) (88.8586, 66.7208) (88.8662, 66.7399) (88.8769, 66.7688) (88.8898, 66.8078) (88.9041, 66.8572) (88.917, 66.9071) (88.929, 66.9573) (88.9407, 67.0077) (88.952, 67.0582) (88.963, 67.1089) (88.9735, 67.1596) (88.9835, 67.2106) (88.9929, 67.2618) (89.0016, 67.3132) (89.0097, 67.3647) (89.0173, 67.4165) (89.0244, 67.4684) (89.0311, 67.5204) (89.0375, 67.5725) (89.0435, 67.6247) (89.0491, 67.6771) (89.0543, 67.7295) (89.0591, 67.7821) (89.0635, 67.8348) (89.0675, 67.8876) (89.0711, 67.9405) (89.0744, 67.9935) (89.0773, 68.0466) (89.0799, 68.0998) (89.0822, 68.1531) (89.0841, 68.2064) (89.0856, 68.2599) (89.0869, 68.3134) (89.0878, 68.367) (89.0884, 68.4207) (89.0886, 68.4745) (89.0886, 68.5283) (89.0882, 68.5822) (89.0875, 68.6362) (89.0865, 68.6903) (89.0852, 68.7444) (89.0837, 68.7985) (89.0818, 68.8528) (89.0796, 68.9071) (89.0771, 68.9615) (89.0744, 69.0159) (89.0713, 69.0704) (89.068, 69.1249) (89.0644, 69.1795) (89.0605, 69.2341) (89.0563, 69.2888) (89.0518, 69.3435) (89.0471, 69.3983) (89.0421, 69.4532) (89.0368, 69.5081) (89.0313, 69.563) (89.0255, 69.618) (89.0194, 69.673) (89.0131, 69.728) (89.0064, 69.7831) (88.9996, 69.8382) (88.9924, 69.8934) (88.9851, 69.9486) (88.9774, 70.0039) (88.9695, 70.0592) (88.9613, 70.1145) (88.9529, 70.1698) (88.9443, 70.2252) (88.9353, 70.2806) (88.9262, 70.336) (88.9186, 70.3804) (88.9129, 70.4137) (88.909, 70.4359) (88.907, 70.447) knots 0 0 0 0 0 0 0.01428571 0.02857143 0.04285714 0.05714286 0.07142857 0.08571429 0.1 0.11428571 0.12857143 0.14285714 0.15714286 0.17142857 0.18571429 0.2 0.21428571 0.22857143 0.24285714 0.25714286 0.27142857 0.28571429 0.3 0.31428571 0.32857143 0.34285714 0.35714286 0.37142857 0.38571429 0.4 0.41428571 0.42857143 0.44285714 0.45714286 0.47142857 0.48571429 0.5 0.51428571 0.52857143 0.54285714 0.55714286 0.57142857 0.58571429 0.6 0.61428571 0.62857143 0.64285714 0.65714286 0.67142857 0.68571429 0.7 0.71428571 0.72857143 0.74285714 0.75714286 0.77142857 0.78571429 0.8 0.81428571 0.82857143 0.84285714 0.85714286 0.87142857 0.88571429 0.9 0.91428571 0.92857143 0.94285714 0.95714286 0.97142857 0.98571429 1 1 1 1 1 1
  arc A48 (88.907, 70.447) -> (87.538, 70.8918) centre (79.882, 45) ccw
  spline S21 degree 5 poles (87.538, 70.8918) (87.5299, 70.884) (87.5137, 70.8683) (87.4895, 70.8448) (87.4573, 70.8133) (87.4173, 70.7738) (87.3775, 70.7343) (87.3379, 70.6945) (87.2986, 70.6547) (87.2595, 70.6148) (87.2206, 70.5747) (87.1819, 70.5345) (87.1435, 70.4942) (87.1053, 70.4537) (87.0673, 70.4132) (87.0296, 70.3725) (86.9921, 70.3317) (86.9549, 70.2907) (86.9179, 70.2497) (86.8811, 70.2085) (86.8446, 70.1672) (86.8083, 70.1258) (86.7722, 70.0842) (86.7365, 70.0426) (86.7009, 70.0008) (86.6657, 69.9589) (86.6307, 69.9168) (86.5959, 69.8747) (86.5614, 69.8324) (86.5272, 69.79) (86.4932, 69.7475) (86.4596, 69.7048) (86.4262, 69.662) (86.393, 69.6191) (86.3602, 69.5761) (86.3276, 69.533) (86.2954, 69.4897) (86.2634, 69.4463) (86.2317, 69.4028) (86.2003, 69.3591) (86.1692, 69.3153) (86.1384, 69.2714) (86.108, 69.2274) (86.0778, 69.1832) (86.048, 69.1389) (86.0185, 69.0945) (85.9893, 69.05) (85.9605, 69.0053) (85.932, 68.9605) (85.9038, 68.9156) (85.876, 68.8705) (85.8486, 68.8253) (85.8216, 68.7799) (85.7949, 68.7344) (85.7687, 68.6888) (85.7429, 68.643) (85.7174, 68.5971) (85.6923, 68.551) (85.6675, 68.5049) (85.6432, 68.4586) (85.6195, 68.4121) (85.5963, 68.3654) (85.5738, 68.3185) (85.5519, 68.2714) (85.5306, 68.2241) (85.5098, 68.1767) (85.4892, 68.1292) (85.469, 68.0816) (85.4493, 68.0339) (85.4304, 67.9859) (85.4129, 67.9375) (85.4004, 67.8984) (85.392, 67.8687) (85.387, 67.8488) (85.3845, 67.8388) knots -1 -1 -1 -1 -1 -1 -0.98571429 -0.97142857 -0.95714286 -0.94285714 -0.92857143 -0.91428571 -0.9 -0.88571429 -0.87142857 -0.85714286 -0.84285714 -0.82857143 -0.81428571 -0.8 -0.78571429 -0.77142857 -0.75714286 -0.74285714 -0.72857143 -0.71428571 -0.7 -0.68571429 -0.67142857 -0.65714286 -0.64285714 -0.62857143 -0.61428571 -0.6 -0.58571429 -0.57142857 -0.55714286 -0.54285714 -0.52857143 -0.51428571 -0.5 -0.48571429 -0.47142857 -0.45714286 -0.44285714 -0.42857143 -0.41428571 -0.4 -0.38571429 -0.37142857 -0.35714286 -0.34285714 -0.32857143 -0.31428571 -0.3 -0.28571429 -0.27142857 -0.25714286 -0.24285714 -0.22857143 -0.21428571 -0.2 -0.18571429 -0.17142857 -0.15714286 -0.14285714 -0.12857143 -0.11428571 -0.1 -0.08571429 -0.07142857 -0.05714286 -0.04285714 -0.02857143 -0.01428571 0 0 0 0 0 0
  line L23 (85.3845, 67.8388) -> (85.2675, 67.3546)
  arc A49 (84.675, 66.9836) -> (85.2675, 67.3546) centre (84.7815, 67.4721) ccw
  arc A50 (84.675, 66.9836) -> (83.5183, 67.2042) centre (79.882, 45) ccw
  arc A51 (83.104, 67.7673) -> (83.5183, 67.2042) centre (83.5991, 67.6976) ccw
  line L24 (83.104, 67.7673) -> (83.1734, 68.2606)
  spline S22 degree 5 poles (83.1734, 68.2606) (83.1749, 68.2708) (83.1775, 68.2912) (83.1806, 68.3218) (83.1834, 68.3628) (83.1849, 68.4142) (83.185, 68.4658) (83.1842, 68.5174) (83.183, 68.5691) (83.1814, 68.6209) (83.1794, 68.6726) (83.177, 68.7244) (83.174, 68.7763) (83.1704, 68.8282) (83.166, 68.8801) (83.161, 68.9321) (83.1555, 68.9841) (83.1495, 69.0361) (83.1431, 69.0882) (83.1363, 69.1402) (83.1291, 69.1923) (83.1215, 69.2444) (83.1135, 69.2965) (83.1051, 69.3486) (83.0963, 69.4008) (83.087, 69.4529) (83.0774, 69.505) (83.0674, 69.5572) (83.057, 69.6094) (83.0462, 69.6615) (83.0352, 69.7137) (83.0238, 69.7658) (83.012, 69.818) (82.9999, 69.8701) (82.9874, 69.9223) (82.9746, 69.9744) (82.9615, 70.0266) (82.9481, 70.0787) (82.9343, 70.1308) (82.9202, 70.1829) (82.9058, 70.2351) (82.8911, 70.2871) (82.8761, 70.3392) (82.8608, 70.3913) (82.8452, 70.4434) (82.8293, 70.4954) (82.8131, 70.5474) (82.7966, 70.5994) (82.7798, 70.6514) (82.7627, 70.7034) (82.7453, 70.7553) (82.7277, 70.8073) (82.7098, 70.8592) (82.6916, 70.9111) (82.6731, 70.963) (82.6543, 71.0148) (82.6353, 71.0666) (82.616, 71.1184) (82.5964, 71.1702) (82.5766, 71.2219) (82.5565, 71.2737) (82.5361, 71.3254) (82.5155, 71.377) (82.4946, 71.4287) (82.4734, 71.4803) (82.452, 71.5318) (82.4304, 71.5834) (82.4085, 71.6349) (82.3863, 71.6864) (82.3639, 71.7378) (82.3412, 71.7892) (82.3229, 71.8303) (82.309, 71.8612) (82.2997, 71.8817) (82.2951, 71.892) knots 0 0 0 0 0 0 0.01428571 0.02857143 0.04285714 0.05714286 0.07142857 0.08571429 0.1 0.11428571 0.12857143 0.14285714 0.15714286 0.17142857 0.18571429 0.2 0.21428571 0.22857143 0.24285714 0.25714286 0.27142857 0.28571429 0.3 0.31428571 0.32857143 0.34285714 0.35714286 0.37142857 0.38571429 0.4 0.41428571 0.42857143 0.44285714 0.45714286 0.47142857 0.48571429 0.5 0.51428571 0.52857143 0.54285714 0.55714286 0.57142857 0.58571429 0.6 0.61428571 0.62857143 0.64285714 0.65714286 0.67142857 0.68571429 0.7 0.71428571 0.72857143 0.74285714 0.75714286 0.77142857 0.78571429 0.8 0.81428571 0.82857143 0.84285714 0.85714286 0.87142857 0.88571429 0.9 0.91428571 0.92857143 0.94285714 0.95714286 0.97142857 0.98571429 1 1 1 1 1 1
  arc A52 (82.2951, 71.892) -> (80.8584, 71.9823) centre (79.882, 45) ccw
  spline S23 degree 5 poles (80.8584, 71.9823) (80.8525, 71.9727) (80.8407, 71.9535) (80.8231, 71.9247) (80.7998, 71.8862) (80.7709, 71.838) (80.7422, 71.7898) (80.7137, 71.7415) (80.6855, 71.6932) (80.6576, 71.6447) (80.6299, 71.5962) (80.6024, 71.5477) (80.5752, 71.4991) (80.5483, 71.4504) (80.5216, 71.4017) (80.4952, 71.3529) (80.469, 71.304) (80.4431, 71.2551) (80.4175, 71.2062) (80.3921, 71.1571) (80.367, 71.108) (80.3421, 71.0589) (80.3176, 71.0097) (80.2933, 70.9604) (80.2693, 70.9111) (80.2455, 70.8618) (80.2221, 70.8123) (80.1989, 70.7629) (80.176, 70.7133) (80.1534, 70.6637) (80.1311, 70.6141) (80.1091, 70.5644) (80.0874, 70.5147) (80.066, 70.4649) (80.0448, 70.4151) (80.024, 70.3652) (80.0035, 70.3152) (79.9833, 70.2652) (79.9635, 70.2152) (79.9439, 70.1651) (79.9247, 70.115) (79.9058, 70.0648) (79.8872, 70.0146) (79.869, 69.9643) (79.8512, 69.914) (79.8336, 69.8636) (79.8165, 69.8132) (79.7996, 69.7628) (79.7831, 69.7123) (79.767, 69.6618) (79.7513, 69.6112) (79.736, 69.5606) (79.7211, 69.5099) (79.7067, 69.4592) (79.6926, 69.4085) (79.679, 69.3577) (79.6657, 69.3069) (79.6528, 69.2561) (79.6404, 69.2052) (79.6283, 69.1543) (79.6169, 69.1034) (79.606, 69.0524) (79.5959, 69.0014) (79.5864, 68.9503) (79.5776, 68.8992) (79.5692, 68.8481) (79.5611, 68.797) (79.5533, 68.7459) (79.5461, 68.6947) (79.5397, 68.6436) (79.5348, 68.5924) (79.5324, 68.5513) (79.5317, 68.5205) (79.5317, 68.5) (79.5319, 68.4897) knots -1 -1 -1 -1 -1 -1 -0.98571429 -0.97142857 -0.95714286 -0.94285714 -0.92857143 -0.91428571 -0.9 -0.88571429 -0.87142857 -0.85714286 -0.84285714 -0.82857143 -0.81428571 -0.8 -0.78571429 -0.77142857 -0.75714286 -0.74285714 -0.72857143 -0.71428571 -0.7 -0.68571429 -0.67142857 -0.65714286 -0.64285714 -0.62857143 -0.61428571 -0.6 -0.58571429 -0.57142857 -0.55714286 -0.54285714 -0.52857143 -0.51428571 -0.5 -0.48571429 -0.47142857 -0.45714286 -0.44285714 -0.42857143 -0.41428571 -0.4 -0.38571429 -0.37142857 -0.35714286 -0.34285714 -0.32857143 -0.31428571 -0.3 -0.28571429 -0.27142857 -0.25714286 -0.24285714 -0.22857143 -0.21428571 -0.2 -0.18571429 -0.17142857 -0.15714286 -0.14285714 -0.12857143 -0.11428571 -0.1 -0.08571429 -0.07142857 -0.05714286 -0.04285714 -0.02857143 -0.01428571 0 0 0 0 0 0
  line L25 (79.5319, 68.4897) -> (79.5389, 67.9916)
  arc A53 (79.0573, 67.4849) -> (79.5389, 67.9916) centre (79.039, 67.9845) ccw
  arc A54 (79.0573, 67.4849) -> (77.8821, 67.4109) centre (79.882, 45) ccw
  arc A55 (77.3408, 67.8533) -> (77.8821, 67.4109) centre (77.8377, 67.909) ccw
  line L26 (77.3408, 67.8533) -> (77.2853, 68.3484)
  spline S24 degree 5 poles (77.2853, 68.3484) (77.2842, 68.3586) (77.2817, 68.379) (77.2771, 68.4095) (77.2696, 68.4499) (77.2583, 68.5) (77.2456, 68.55) (77.232, 68.5998) (77.2179, 68.6496) (77.2034, 68.6993) (77.1887, 68.7489) (77.1735, 68.7985) (77.1577, 68.848) (77.1413, 68.8973) (77.1241, 68.9466) (77.1064, 68.9957) (77.0881, 69.0447) (77.0693, 69.0936) (77.0501, 69.1424) (77.0306, 69.1911) (77.0107, 69.2398) (76.9904, 69.2884) (76.9697, 69.3368) (76.9486, 69.3852) (76.9271, 69.4335) (76.9051, 69.4817) (76.8828, 69.5298) (76.8602, 69.5779) (76.8371, 69.6258) (76.8138, 69.6736) (76.7901, 69.7214) (76.766, 69.7691) (76.7417, 69.8167) (76.717, 69.8642) (76.6919, 69.9116) (76.6666, 69.9589) (76.6409, 70.0062) (76.6149, 70.0533) (76.5886, 70.1004) (76.562, 70.1474) (76.5351, 70.1942) (76.5079, 70.241) (76.4804, 70.2878) (76.4527, 70.3344) (76.4246, 70.3809) (76.3962, 70.4274) (76.3676, 70.4737) (76.3387, 70.52) (76.3095, 70.5662) (76.28, 70.6123) (76.2503, 70.6583) (76.2203, 70.7042) (76.19, 70.75) (76.1595, 70.7957) (76.1287, 70.8414) (76.0976, 70.8869) (76.0663, 70.9324) (76.0347, 70.9778) (76.0029, 71.0231) (75.9708, 71.0682) (75.9385, 71.1133) (75.9059, 71.1583) (75.8731, 71.2033) (75.84, 71.2481) (75.8067, 71.2928) (75.7731, 71.3374) (75.7393, 71.382) (75.7053, 71.4264) (75.671, 71.4708) (75.6365, 71.515) (75.6017, 71.5592) (75.5738, 71.5944) (75.5527, 71.6208) (75.5386, 71.6384) (75.5315, 71.6472) knots 0 0 0 0 0 0 0.01428571 0.02857143 0.04285714 0.05714286 0.07142857 0.08571429 0.1 0.11428571 0.12857143 0.14285714 0.15714286 0.17142857 0.18571429 0.2 0.21428571 0.22857143 0.24285714 0.25714286 0.27142857 0.28571429 0.3 0.31428571 0.32857143 0.34285714 0.35714286 0.37142857 0.38571429 0.4 0.41428571 0.42857143 0.44285714 0.45714286 0.47142857 0.48571429 0.5 0.51428571 0.52857143 0.54285714 0.55714286 0.57142857 0.58571429 0.6 0.61428571 0.62857143 0.64285714 0.65714286 0.67142857 0.68571429 0.7 0.71428571 0.72857143 0.74285714 0.75714286 0.77142857 0.78571429 0.8 0.81428571 0.82857143 0.84285714 0.85714286 0.87142857 0.88571429 0.9 0.91428571 0.92857143 0.94285714 0.95714286 0.97142857 0.98571429 1 1 1 1 1 1
  arc A56 (75.5315, 71.6472) -> (74.1175, 71.3775) centre (79.882, 45) ccw
  spline S25 degree 5 poles (74.1175, 71.3775) (74.1142, 71.3667) (74.1076, 71.3452) (74.0977, 71.3129) (74.0846, 71.2698) (74.0686, 71.2159) (74.0528, 71.1621) (74.0372, 71.1082) (74.022, 71.0544) (74.0069, 71.0005) (73.9922, 70.9467) (73.9776, 70.8928) (73.9634, 70.839) (73.9494, 70.7851) (73.9357, 70.7313) (73.9222, 70.6775) (73.909, 70.6236) (73.8961, 70.5698) (73.8834, 70.516) (73.8711, 70.4622) (73.8589, 70.4084) (73.8471, 70.3546) (73.8355, 70.3009) (73.8243, 70.2471) (73.8133, 70.1934) (73.8026, 70.1397) (73.7921, 70.086) (73.782, 70.0323) (73.7721, 69.9786) (73.7626, 69.925) (73.7533, 69.8713) (73.7443, 69.8177) (73.7357, 69.7642) (73.7273, 69.7106) (73.7193, 69.6571) (73.7115, 69.6036) (73.7041, 69.5501) (73.697, 69.4967) (73.6901, 69.4433) (73.6837, 69.3899) (73.6775, 69.3366) (73.6717, 69.2833) (73.6662, 69.23) (73.6611, 69.1768) (73.6563, 69.1236) (73.6518, 69.0705) (73.6477, 69.0174) (73.644, 68.9643) (73.6406, 68.9113) (73.6375, 68.8584) (73.6349, 68.8055) (73.6326, 68.7527) (73.6308, 68.6999) (73.6294, 68.6472) (73.6284, 68.5946) (73.6278, 68.542) (73.6276, 68.4895) (73.6278, 68.4371) (73.6283, 68.3847) (73.6294, 68.3324) (73.6309, 68.2802) (73.6331, 68.2281) (73.636, 68.1762) (73.6395, 68.1244) (73.6436, 68.0727) (73.6482, 68.0211) (73.6531, 67.9696) (73.6583, 67.9181) (73.664, 67.8668) (73.6705, 67.8156) (73.6785, 67.7648) (73.6864, 67.7245) (73.6934, 67.6945) (73.6985, 67.6746) (73.7012, 67.6647) knots -1 -1 -1 -1 -1 -1 -0.98571429 -0.97142857 -0.95714286 -0.94285714 -0.92857143 -0.91428571 -0.9 -0.88571429 -0.87142857 -0.85714286 -0.84285714 -0.82857143 -0.81428571 -0.8 -0.78571429 -0.77142857 -0.75714286 -0.74285714 -0.72857143 -0.71428571 -0.7 -0.68571429 -0.67142857 -0.65714286 -0.64285714 -0.62857143 -0.61428571 -0.6 -0.58571429 -0.57142857 -0.55714286 -0.54285714 -0.52857143 -0.51428571 -0.5 -0.48571429 -0.47142857 -0.45714286 -0.44285714 -0.42857143 -0.41428571 -0.4 -0.38571429 -0.37142857 -0.35714286 -0.34285714 -0.32857143 -0.31428571 -0.3 -0.28571429 -0.27142857 -0.25714286 -0.24285714 -0.22857143 -0.21428571 -0.2 -0.18571429 -0.17142857 -0.15714286 -0.14285714 -0.12857143 -0.11428571 -0.1 -0.08571429 -0.07142857 -0.05714286 -0.04285714 -0.02857143 -0.01428571 0 0 0 0 0 0
  line L27 (73.7012, 67.6647) -> (73.8319, 67.184)
  arc A57 (73.4915, 66.5734) -> (73.8319, 67.184) centre (73.3494, 67.0528) ccw
  arc A58 (73.4915, 66.5734) -> (72.3716, 66.2095) centre (79.882, 45) ccw
  arc A59 (71.7372, 66.5034) -> (72.3716, 66.2095) centre (72.2047, 66.6808) ccw
  line L28 (71.7372, 66.5034) -> (71.5604, 66.9691)
  spline S26 degree 5 poles (71.5604, 66.9691) (71.5568, 66.9787) (71.5492, 66.9978) (71.5372, 67.0262) (71.5199, 67.0635) (71.4965, 67.1092) (71.4718, 67.1545) (71.4462, 67.1993) (71.4202, 67.244) (71.3938, 67.2886) (71.3672, 67.333) (71.3401, 67.3773) (71.3125, 67.4213) (71.2843, 67.465) (71.2555, 67.5084) (71.2261, 67.5515) (71.1962, 67.5944) (71.1658, 67.6371) (71.1351, 67.6796) (71.1041, 67.722) (71.0727, 67.7642) (71.041, 67.8062) (71.0089, 67.848) (70.9764, 67.8896) (70.9435, 67.931) (70.9103, 67.9723) (70.8767, 68.0133) (70.8428, 68.0542) (70.8086, 68.0949) (70.7741, 68.1354) (70.7392, 68.1758) (70.7041, 68.216) (70.6687, 68.256) (70.6329, 68.2959) (70.5969, 68.3356) (70.5606, 68.3751) (70.5239, 68.4145) (70.487, 68.4537) (70.4499, 68.4928) (70.4124, 68.5317) (70.3747, 68.5704) (70.3367, 68.6089) (70.2985, 68.6474) (70.26, 68.6856) (70.2212, 68.7237) (70.1822, 68.7616) (70.143, 68.7994) (70.1034, 68.837) (70.0637, 68.8745) (70.0237, 68.9118) (69.9834, 68.949) (69.943, 68.986) (69.9022, 69.0229) (69.8613, 69.0596) (69.8201, 69.0961) (69.7787, 69.1325) (69.737, 69.1688) (69.6952, 69.2048) (69.6531, 69.2408) (69.6108, 69.2766) (69.5682, 69.3122) (69.5255, 69.3477) (69.4825, 69.383) (69.4393, 69.4182) (69.3959, 69.4533) (69.3523, 69.4881) (69.3085, 69.5229) (69.2645, 69.5575) (69.2203, 69.5919) (69.1759, 69.6262) (69.1312, 69.6603) (69.0954, 69.6875) (69.0684, 69.7078) (69.0503, 69.7213) (69.0413, 69.7281) knots 0 0 0 0 0 0 0.01428571 0.02857143 0.04285714 0.05714286 0.07142857 0.08571429 0.1 0.11428571 0.12857143 0.14285714 0.15714286 0.17142857 0.18571429 0.2 0.21428571 0.22857143 0.24285714 0.25714286 0.27142857 0.28571429 0.3 0.31428571 0.32857143 0.34285714 0.35714286 0.37142857 0.38571429 0.4 0.41428571 0.42857143 0.44285714 0.45714286 0.47142857 0.48571429 0.5 0.51428571 0.52857143 0.54285714 0.55714286 0.57142857 0.58571429 0.6 0.61428571 0.62857143 0.64285714 0.65714286 0.67142857 0.68571429 0.7 0.71428571 0.72857143 0.74285714 0.75714286 0.77142857 0.78571429 0.8 0.81428571 0.82857143 0.84285714 0.85714286 0.87142857 0.88571429 0.9 0.91428571 0.92857143 0.94285714 0.95714286 0.97142857 0.98571429 1 1 1 1 1 1
  arc A60 (69.0413, 69.7281) -> (67.7388, 69.1152) centre (79.882, 45) ccw